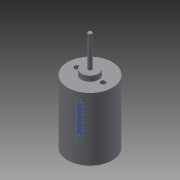
# Autodesk Inventor part: motor
Saved by Autodesk Inventor 2015 (Build 190159000, 159)
## iProperties
Created: 2015-12-08
Part Number: motor
Material: Generic
Document SubType Name: Modeling
Designer: boztalay
Density: 1 g/cm^3
Appearance: Default
Author: boztalay
Autodesk Inventor part; units mm, degrees
ref_plane "YZ Plane" through (0, 0, 0) normal (1, 0, 0) x (0, 1, 0)
ref_plane "XZ Plane" through (0, 0, 0) normal (0, 1, 0) x (-1, 0, 0)
ref_plane "XY Plane" through (0, 0, 0) normal (0, 0, 1) x (1, 0, 0)
sketch "Sketch1" plane through (0, 0, 0) normal (0, 1, 0) x (-1, 0, 0)
  circle A0 centre (0, 0) radius 13.4938
  dimension "d0" = 26.9875
  constraints: 1 centre point, 1 coincident
  measures "d0" diameter of A0
extrude "Extrusion1" add sketch "Sketch1" along normal blind 38.1
sketch "Sketch2" plane through (0, 38.1, 0) normal (0, 1, 0) x (1, 0, 0)
  circle A0 centre (0, 0) radius 5.1594
  dimension "d3" = 10.3187
  constraints: 1 centre point, 1 coincident
  measures "d3" diameter of A0
extrude "Extrusion2" add sketch "Sketch2" along normal blind 3.175
sketch "Sketch3" plane through (0, 38.1, 0) normal (0, 1, 0) x (1, 0, 0)
  circle A0 centre (-7.9375, 0) radius 1.524
  line L0 (0, 0) -> (-7.9375, 0) construction
  line L1 (0, -15.84) -> (0, 17.6643) construction
  circle A1 centre (7.9375, 0) radius 1.524
  line L2 (0, 0) -> (7.9375, 0) construction
  dimension "d6" = 3.048
  dimension "d7" = 7.9375
  dimension "d8" = 0
  dimension "d9" = 17.6643
  dimension "d10" = 15.8399
  constraints: 6 end point, 2 centre point, 1 horizontal, 1 symmetric about line, 1 vertical, 1 other
  measures "d6" diameter of A0
  measures "d7" distance of L0.start L0.end
  measures "d8" distance from line of L0.start L1
  measures "d9" distance from line of L1.end L0
  measures "d10" distance from line of L1.start L0
extrude "Extrusion3" cut sketch "Sketch3" against normal blind 3.175
sketch "Sketch6" plane through (0, 41.275, 0) normal (0, 1, 0) x (1, 0, 0)
  circle A0 centre (0, 0) radius 1.1557
  dimension "d18" = 2.3114
  constraints: 1 centre point, 1 coincident
  measures "d18" diameter of A0
extrude "Extrusion6" add sketch "Sketch6" along normal blind 19.05
body "Solid1"
